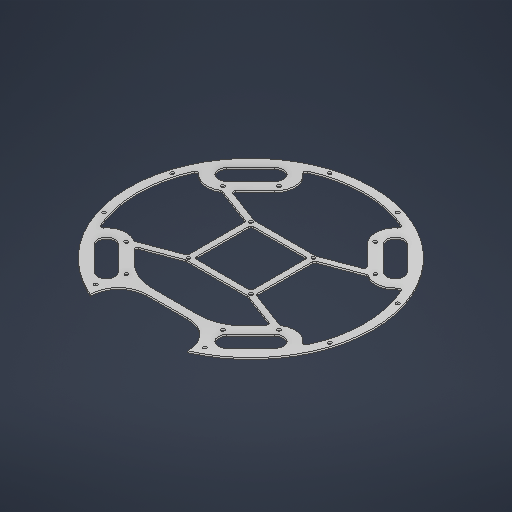
# Autodesk Inventor part: TopCarbonRing-WithoutClosure
Saved by Autodesk Inventor 2025.2 (Build 292293000, 293)
## iProperties
Created: 2023-05-12
Part Number: TopCarbonRing-WithoutClosure
Material: Aluminum 6061
Document SubType Name: Modeling
Designer: Elias Braun
Density: 2.7 g/cm^3
Appearance: Aluminum - Polished
Author: Elias Braun
Autodesk Inventor part; units mm, degrees
ref_plane "YZ Plane" through (0, 0, 0) normal (1, 0, 0) x (0, 1, 0)
ref_plane "XZ Plane" through (0, 0, 0) normal (0, 1, 0) x (-1, 0, 0)
ref_plane "XY Plane" through (0, 0, 0) normal (0, 0, 1) x (1, 0, 0)
sketch "Sketch1" plane through (0, 0, 0) normal (0, 1, 0) x (-1, 0, 0)
  line L0 (-57.9025, 44.628) -> (-43.0581, 59.4724)
  arc A0 (-17.5, 66.5) -> (-43.0581, 59.4724) centre (-19.5145, 23.8377) ccw
  line L1 (-17.5, 66.5) -> (18.0581, 66.5)
  arc A1 (44.5267, 58.0038) -> (18.0581, 66.5) centre (19.5089, 25.5422) ccw
  line L2 (44.5267, 58.0038) -> (57.9025, 44.628)
  arc A2 (57.1925, 41.3419) -> (57.9025, 44.628) centre (56.4883, 43.2138) ccw
  line L3 (57.1925, 41.3419) -> (27.3858, 30.1281)
  arc A3 (26.6815, 30) -> (27.3858, 30.1281) centre (26.6815, 32) ccw
  line L4 (26.6815, 30) -> (-26.6815, 30)
  arc A4 (-27.3858, 30.1281) -> (-26.6815, 30) centre (-26.6815, 32) ccw
  line L5 (-27.3858, 30.1281) -> (-57.1925, 41.3419)
  arc A5 (-57.9025, 44.628) -> (-57.1925, 41.3419) centre (-56.4883, 43.2138) ccw
  line L6 (-63.3138, 38.3027) -> (-31.2958, 26.257)
  arc A6 (-30, 24.385) -> (-31.2958, 26.257) centre (-32, 24.385) ccw
  line L7 (-30, 24.385) -> (-30, -24.385)
  arc A7 (-31.2958, -26.257) -> (-30, -24.385) centre (-32, -24.385) ccw
  line L8 (-31.2958, -26.257) -> (-63.3138, -38.3027)
  arc A8 (-65.0671, -38.1335) -> (-63.3138, -38.3027) centre (-64.0181, -36.4307) ccw
  arc A9 (-65.0671, -38.1335) -> (-87.6848, -41.8234) centre (-74.2462, -53.033) ccw
  arc A10 (-91.0415, -41.3697) -> (-87.6848, -41.8234) centre (-89.2206, -40.5423) ccw
  arc A11 (-91.0415, 41.3697) -> (-91.0415, -41.3697) centre (0, 0) ccw
  arc A12 (-87.6848, 41.8234) -> (-91.0415, 41.3697) centre (-89.2206, 40.5423) ccw
  arc A13 (-87.6848, 41.8234) -> (-65.0671, 38.1335) centre (-74.2462, 53.033) ccw
  arc A14 (-63.3138, 38.3027) -> (-65.0671, 38.1335) centre (-64.0181, 36.4307) ccw
  line L9 (-57.1925, -41.3419) -> (-27.3858, -30.1281)
  arc A15 (-26.6815, -30) -> (-27.3858, -30.1281) centre (-26.6815, -32) ccw
  line L10 (-26.6815, -30) -> (26.6815, -30)
  arc A16 (27.3858, -30.1281) -> (26.6815, -30) centre (26.6815, -32) ccw
  line L11 (27.3858, -30.1281) -> (57.1925, -41.3419)
  arc A17 (57.9025, -44.628) -> (57.1925, -41.3419) centre (56.4883, -43.2138) ccw
  line L12 (57.9025, -44.628) -> (40.6586, -61.8718)
  arc A18 (40.6586, -61.8718) -> (41.8234, -87.6848) centre (53.033, -74.2462) ccw
  arc A19 (41.3697, -91.0415) -> (41.8234, -87.6848) centre (40.5423, -89.2206) ccw
  arc A20 (-41.3697, -91.0415) -> (41.3697, -91.0415) centre (0, 0) ccw
  arc A21 (-41.8234, -87.6848) -> (-41.3697, -91.0415) centre (-40.5423, -89.2206) ccw
  arc A22 (-41.8234, -87.6848) -> (-40.6586, -61.8718) centre (-53.033, -74.2462) ccw
  line L13 (-40.6586, -61.8718) -> (-57.9025, -44.628)
  arc A23 (-57.1925, -41.3419) -> (-57.9025, -44.628) centre (-56.4883, -43.2138) ccw
  line L14 (23, -25) -> (-23, -25)
  arc A24 (-25, -23) -> (-23, -25) centre (-23, -23) ccw
  line L15 (-25, -23) -> (-25, 23)
  arc A25 (-23, 25) -> (-25, 23) centre (-23, 23) ccw
  line L16 (-23, 25) -> (23, 25)
  arc A26 (25, 23) -> (23, 25) centre (23, 23) ccw
  line L17 (25, 23) -> (25, -23)
  arc A27 (23, -25) -> (25, -23) centre (23, -23) ccw
  line L18 (63.3138, -38.3027) -> (31.2958, -26.257)
  arc A28 (30, -24.385) -> (31.2958, -26.257) centre (32, -24.385) ccw
  line L19 (30, -24.385) -> (30, 24.385)
  arc A29 (31.2958, 26.257) -> (30, 24.385) centre (32, 24.385) ccw
  line L20 (31.2958, 26.257) -> (63.3138, 38.3027)
  arc A30 (65.0671, 38.1335) -> (63.3138, 38.3027) centre (64.0181, 36.4307) ccw
  arc A31 (65.0671, 38.1335) -> (87.6848, 41.8234) centre (74.2462, 53.033) ccw
  arc A32 (91.0415, 41.3697) -> (87.6848, 41.8234) centre (89.2206, 40.5423) ccw
  arc A33 (91.0415, -41.3697) -> (91.0415, 41.3697) centre (0, 0) ccw
  arc A34 (87.6848, -41.8234) -> (91.0415, -41.3697) centre (89.2206, -40.5423) ccw
  arc A35 (87.6848, -41.8234) -> (65.0671, -38.1335) centre (74.2462, -53.033) ccw
  arc A36 (63.3138, -38.3027) -> (65.0671, -38.1335) centre (64.0181, -36.4307) ccw
  arc A37 (-43.0581, 98.5) -> (-18.0581, 73.5) centre (-18.0581, 98.5) ccw
  arc A38 (-43.0581, 98.5) -> (43.0581, 98.5) centre (0, 0) ccw
  arc A39 (18.0581, 73.5) -> (43.0581, 98.5) centre (18.0581, 98.5) ccw
  line L21 (18.0581, 73.5) -> (-18.0581, 73.5)
  arc A40 (-68.9429, -47.7297) -> (-79.5495, -58.3363) centre (-74.2462, -53.033) ccw
  line L22 (-68.9429, -47.7297) -> (-47.7297, -68.9429)
  arc A41 (-58.3363, -79.5495) -> (-47.7297, -68.9429) centre (-53.033, -74.2462) ccw
  line L23 (-58.3363, -79.5495) -> (-79.5495, -58.3363)
  arc A42 (-47.7297, 68.9429) -> (-58.3363, 79.5495) centre (-53.033, 74.2462) ccw
  line L24 (-47.7297, 68.9429) -> (-68.9429, 47.7297)
  arc A43 (-79.5495, 58.3363) -> (-68.9429, 47.7297) centre (-74.2462, 53.033) ccw
  line L25 (-79.5495, 58.3363) -> (-58.3363, 79.5495)
  arc A44 (68.9429, 47.7297) -> (79.5495, 58.3363) centre (74.2462, 53.033) ccw
  line L26 (68.9429, 47.7297) -> (47.7297, 68.9429)
  arc A45 (58.3363, 79.5495) -> (47.7297, 68.9429) centre (53.033, 74.2462) ccw
  line L27 (58.3363, 79.5495) -> (79.5495, 58.3363)
  arc A46 (47.7297, -68.9429) -> (58.3363, -79.5495) centre (53.033, -74.2462) ccw
  line L28 (47.7297, -68.9429) -> (68.9429, -47.7297)
  arc A47 (79.5495, -58.3363) -> (68.9429, -47.7297) centre (74.2462, -53.033) ccw
  line L29 (79.5495, -58.3363) -> (58.3363, -79.5495)
  circle A48 centre (-27.5, 27.5) radius 1.6
  circle A49 centre (27.5, 27.5) radius 1.6
  circle A50 centre (-27.5, -27.5) radius 1.6
  circle A51 centre (27.5, -27.5) radius 1.6
  circle A52 centre (-67.1751, 42.4264) radius 1.6
  circle A53 centre (-67.1751, -42.4264) radius 1.6
  circle A54 centre (67.1751, -42.4264) radius 1.6
  circle A55 centre (67.1751, 42.4264) radius 1.6
  circle A56 centre (30, -99.318) radius 1.6
  circle A57 centre (-99.318, 30) radius 1.6
  circle A58 centre (99.318, 30) radius 1.6
  circle A59 centre (-30, -99.318) radius 1.6
  circle A60 centre (-99.318, -30) radius 1.6
  circle A61 centre (99.318, -30) radius 1.6
  circle A62 centre (48.0581, 88.5) radius 1.6
  circle A63 centre (-48.0581, 88.5) radius 1.6
  circle A64 centre (-42.4264, -67.1751) radius 1.6
  circle A65 centre (-42.4264, 67.1751) radius 1.6
  circle A66 centre (42.4264, 67.1751) radius 1.6
  circle A67 centre (42.4264, -67.1751) radius 1.6
  point P0 (-18.0581, 73.5)
  point P1 (-43.0581, 98.5)
  point P2 (43.0581, 98.5)
  point P3 (-79.5495, -58.3363)
  point P4 (58.3363, 79.5495)
  point P5 (-68.9429, 47.7297)
  point P6 (-79.5495, 58.3363)
  point P7 (65.0671, 38.1335)
  point P8 (91.0415, 41.3697)
  point P9 (91.0415, -41.3697)
  point P10 (31.2958, -26.257)
  point P11 (30, -24.385)
  point P12 (-65.0671, -38.1335)
  point P13 (-91.0415, 41.3697)
  point P14 (-65.0671, 38.1335)
  point P15 (-31.2958, 26.257)
  point P16 (57.9025, -44.628)
  point P17 (41.3697, -91.0415)
  point P18 (-25, -23)
  point P19 (26.6815, 30)
  constraints: 96 point on circle, 68 centre point, 60 end point
extrude "Extrusion1" add sketch "Sketch1" along normal blind 1.5
body "Solid1"
